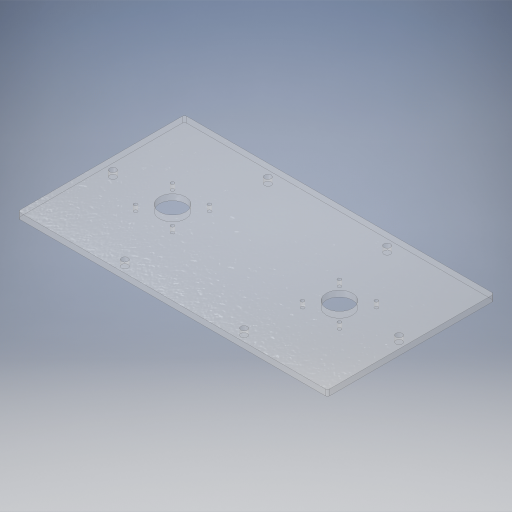
# Autodesk Inventor part: BT001_trajan20_21
Saved by Autodesk Inventor 2023 (Build 270158000, 158)
## iProperties
Company: HTBLA Kaindorf
RuleStatus: InUse
Created: 2022-08-03
Part Number: BT001_trajan20_21
Project: Zeichenmaschine_v2
Material: Acryl
Description: Platte Stepper Motoren
Document SubType Name: Modeling
Designer: trajan20
Density: 1.188 g/cm^3
Appearance: Transparent - farblos
Mass: 210.497 g
Surface Area: 764.437 cm^2
Volume: 177.186 cm^3
AfterDocNew0: iProperties-Editor_aufrufen
Author: jan
Keywords: 2021
Autodesk Inventor part; units mm, degrees
ref_plane "YZ Plane" through (0, 0, 0) normal (1, 0, 0) x (0, 1, 0)
ref_plane "XZ Plane" through (0, 0, 0) normal (0, 1, 0) x (-1, 0, 0)
ref_plane "XY Plane" through (0, 0, 0) normal (0, 0, 1) x (1, 0, 0)
derived "BT000_trajan20_22_Zeichenmaschine_neu_Masterskizze.ipt"
sketch "Skizze3" plane through (0, 0, 0) normal (0, 0, 1) x (1, 0, 0)
  line L0 (0, 0) -> (-140, 0)
  line L1 (-140, 0) -> (-140, 130)
  line L2 (-140, 260) -> (0, 260)
  line L3 (0, 260) -> (0, 0)
  line L4 (-54.5, 44.5) -> (-85.5, 44.5) construction
  line L5 (-54.5, 75.5) -> (-85.5, 75.5) construction
  line L6 (-85.5, 75.5) -> (-85.5, 44.5) construction
  line L7 (-54.5, 75.5) -> (-54.5, 44.5) construction
  circle A0 centre (-70, 60) radius 11
  circle A1 centre (-85.5, 75.5) radius 1.5
  circle A2 centre (-85.5, 44.5) radius 1.5
  circle A3 centre (-54.5, 44.5) radius 1.5
  circle A4 centre (-54.5, 75.5) radius 1.5
  line L8 (-140, 130) -> (-140, 260)
  point P0 (-70, 0)
  point P1 (-70, 10)
  point P2 (-130, 80)
  point P3 (-10, 80)
  dimension "d4" = 260
  dimension "d5" = 140
  dimension "d6" = 31
  dimension "d7" = 31
  dimension "d8" = 15.5
  dimension "d9" = 15.5
  dimension "d10" = 60
  dimension "d11" = 22
  dimension "d12" = 3
  dimension "d13" = 3
  dimension "d14" = 3
  dimension "d15" = 3
  dimension "d22" = 10
  dimension "d23" = 10
  dimension "d26" = 10
  dimension "d57" = 80
  constraints: 26 end point, 5 centre point, 5 coincident, 3 horizontal, 3 parallel, 2 perpendicular, 2 vertical, 2 vertical alignment, 1 horizontal alignment, 1 midpoint
  measures "d4" distance between parallel lines of L2 L0
  measures "d5" distance between parallel lines of L1 L3
  measures "d6" distance between parallel lines of L6 L7
  measures "d7" distance between parallel lines of L5 L4
  measures "d8" distance from line of L7 point (-70, 60)
  measures "d9" distance from line of L5 point (-70, 60)
  measures "d10" distance from line of L0 point (-70, 60)
  measures "d11" diameter of A0
  measures "d12" diameter of A3
  measures "d13" diameter of A2
  measures "d14" diameter of A4
  measures "d15" diameter of A1
  measures "d22" distance from line of L0 point (-70, 10)
  measures "d23" distance from line of point (-10, 80) L3
  measures "d26" distance from line of L1 point (-130, 80)
  measures "d57" distance from line of L0 point (-130, 80)
extrude "Extrusion3" add sketch "Skizze3" against normal blind 5 contours L0 L1 L8 L2 L3 | A0 | A1 | A2 | A3 | A4
fillet "Rundung1" radius 2 4 edges at (0, 0, -2.5) (0, 260, -2.5) (-140, 260, -2.5) (-140, 0, -2.5)
hole "Bohrung1" at (-70, 10, 0) at (-130, 80, 0) at (-10, 80, 0) direction (0, 0, -1) diameter 5.5 end through all
ref_plane "Arbeitsebene3" through (0, 130, 0) normal (0, 1, 0) x (-1, 0, 0)
extrude "Extrusion6" cut sketch "Skizze3" against normal through all contours A0 | A1 | A2 | A3 | A4
mirror "Spiegeln2" about plane through (0, 130, 0) normal (0, 1, 0) of "Extrusion6", "Bohrung1"
equation "\"d8\" = 0.5 * d6"
equation "\"d9\" = d8"
equation "\"d23\" = d22"
equation "\"d26\" = d25"
equation "\"d25\" = d22"
